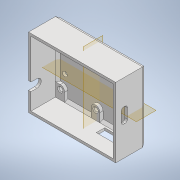
# Autodesk Inventor part: корпус
Saved by Autodesk Inventor 2021 (Build 250183000, 183)
## iProperties
Created: 2024-05-10
Part Number: корпус
Material: Типовые
Document SubType Name: Modeling
Designer: Мария
Density: 1 g/cm^3
Appearance: По умолчанию
Author: Мария
Autodesk Inventor part; units mm, degrees
ref_plane "YZ Plane" through (0, 0, 0) normal (1, 0, 0) x (0, 1, 0)
ref_plane "XZ Plane" through (0, 0, 0) normal (0, 1, 0) x (-1, 0, 0)
ref_plane "XY Plane" through (0, 0, 0) normal (0, 0, 1) x (1, 0, 0)
sketch "Эскиз1" plane through (0, 0, 0) normal (0, 0, 1) x (1, 0, 0)
  line L0 (2, 41.195) -> (54.5, 41.195) projected
  line L1 (54.5, 41.195) -> (54.5, 3.195) projected
  line L2 (0, 0) -> (56.5, 0)
  line L3 (56.5, 0) -> (56.5, 45.2)
  line L4 (56.5, 45.2) -> (0, 45.2)
  line L5 (0, 45.2) -> (0, 0)
  dimension "d0" = 52.5
  dimension "d1" = 38
  dimension "d2" = 56.5
  dimension "d3" = 45.2
  constraints: 8 end point, 2 parallel, 1 horizontal, 1 perpendicular
  measures "d0" distance of L0.start L0.end
  measures "d1" distance of L0.end L1.end
  measures "d2" distance of L3.end L4.end
  measures "d3" distance of L2.end L3.end
extrude "Выдавливание1" add sketch "Эскиз1" along normal blind 1.6
sketch "Эскиз2" plane through (0, 0, 1.6) normal (0, 0, 1) x (1, 0, 0)
  line L0 (56.5, 45.2) -> (0, 45.2) projected
  line L1 (0, 45.2) -> (0, 0) projected
  line L2 (56.5, 0) -> (56.5, 45.2) projected
  line L3 (0, 0) -> (56.5, 0) projected
  line L4 (1.6, 43.6) -> (54.9, 43.6)
  line L5 (54.9, 43.6) -> (54.9, 1.6)
  line L6 (54.9, 1.6) -> (1.6, 1.6)
  line L7 (1.6, 1.6) -> (1.6, 43.6)
  dimension "d6" = 1.6
  dimension "d7" = 1.6
  dimension "d8" = 1.6
  dimension "d9" = 1.6
  constraints: 8 end point, 2 parallel, 1 horizontal, 1 perpendicular
  measures "d6" distance between parallel lines of L0 L4
  measures "d7" distance between parallel lines of L1 L7
  measures "d8" distance between parallel lines of L3 L6
  measures "d9" distance between parallel lines of L2 L5
extrude "Выдавливание2" add sketch "Эскиз2" along normal blind 17.8
ref_plane "РабПлоскость1" through (0, 22.6, 0) normal (0, 1, 0) x (1, 0, 0)
ref_plane "РабПлоскость2" through (28.25, 0, 0) normal (1, 0, 0) x (0, 0, -1)
sketch "Эскиз3" plane through (0, 0, 0) normal (-1, 0, 0) x (0, 0, 1)
  circle A0 centre (15.47, 15.2304) radius 2.7
  line L0 (15.47, 17.9304) -> (19.4, 17.9304)
  line L1 (19.4, 1.6) -> (19.4, 43.6) projected
  line L2 (19.4, 17.9304) -> (19.4, 12.5304)
  line L3 (19.4, 12.5304) -> (15.47, 12.5304)
  line L4 (0, 0) -> (19.4, 0) projected
  circle A1 centre (15.27, 15.2304) radius 2.3 projected
  dimension "d39" = 5.4
  dimension "d41" = 3.93
  constraints: 6 end point, 2 point on circle, 2 point on line, 2 vertical alignment, 1 centre point, 1 horizontal, 1 horizontal alignment, 1 tangent
  measures "d39" diameter of A0
  measures "d41" distance from line of L2 A0.centre
extrude "Выдавливание3" cut sketch "Эскиз3" against normal up to surface (1.6 mm away) contours A0 | A0 L0 L1 L3 | A1
sketch "Эскиз4" plane through (54.9, 1.6, 1.6) normal (-1, 0, 0) x (0, 0, 1)
  line L0 (0, 0) -> (17.8, 0) projected
  line L1 (0, 0) -> (0, 42) projected
  line L2 (12.56, 18.055) -> (11.85, 18.055) projected
  line L3 (11.85, 17.905) -> (12.56, 17.905) projected
  line L4 (12.56, 18.055) -> (11.85, 18.055) projected
  line L5 (11.85, 17.905) -> (12.56, 17.905) projected
  arc A0 (12.56, 17.905) -> (13.81, 19.155) centre (12.56, 19.155) ccw projected
  line L6 (13.81, 19.155) -> (13.81, 25.595) projected
  arc A1 (10.6, 19.155) -> (11.85, 17.905) centre (11.85, 19.155) ccw projected
  line L7 (10.6, 25.595) -> (10.6, 19.155) projected
  arc A2 (11.85, 26.845) -> (10.6, 25.595) centre (11.85, 25.595) ccw projected
  line L8 (12.56, 26.845) -> (11.85, 26.845) projected
  arc A3 (13.81, 25.595) -> (12.56, 26.845) centre (12.56, 25.595) ccw projected
  line L9 (14.21, 25.595) -> (14.21, 19.155)
  arc A4 (12.56, 17.505) -> (14.21, 19.155) centre (12.56, 19.155) ccw
  line L10 (12.56, 17.505) -> (11.85, 17.505)
  arc A5 (10.2, 19.155) -> (11.85, 17.505) centre (11.85, 19.155) ccw
  line L11 (10.2, 19.155) -> (10.2, 25.595)
  arc A6 (11.85, 27.245) -> (10.2, 25.595) centre (11.85, 25.595) ccw
  line L12 (11.85, 27.245) -> (12.56, 27.245)
  arc A7 (14.21, 25.595) -> (12.56, 27.245) centre (12.56, 25.595) ccw
  point P0 (-1.6, -1.6)
  dimension "d50" = 1.65
  constraints: 8 end point, 8 point on circle, 8 tangent, 4 centre point, 3 parallel
  measures "d50" radius of A7
extrude "Выдавливание4" cut sketch "Эскиз4" against normal up to surface (1.6 mm away) contours A1 L7 A2 L8 A3 L6 A0 L3 | L9 A4 L10 A5 L11 A6 L12 A7
sketch "Эскиз5" plane through (0, 0, 0) normal (0, 0, -1) x (-1, 0, 0)
  circle A0 centre (-4.77, 37.84) radius 1.25
  circle A1 centre (-4.77, 7.36) radius 1.25
  circle A2 centre (-51.9, 37.84) radius 1.25
  circle A3 centre (-51.9, 7.36) radius 1.25
  circle A4 centre (-27.63, 37.84) radius 1.25
  circle A5 centre (-27.63, 7.36) radius 1.25
  line L0 (-56.5, 45.2) -> (0, 45.2) projected
  line L1 (0, 0) -> (-56.5, 0) projected
  line L2 (-28.25, -9.04) -> (-28.25, 54.24) projected
  line L3 (-56.5, 0) -> (-56.5, 45.2) projected
  line L4 (0, 45.2) -> (0, 0) projected
  dimension "d22" = 2.5
  dimension "d23" = 2.5
  dimension "d24" = 2.5
  dimension "d25" = 2.5
  dimension "d26" = 2.5
  dimension "d27" = 2.5
  dimension "d43" = 30.48
  dimension "d44" = 45.2
  dimension "d45" = 7.36
  dimension "d47" = 0.62
  dimension "d48" = 4.6
  dimension "d49" = 4.77
  constraints: 6 centre point, 4 horizontal alignment, 3 vertical alignment
  measures "d22" diameter of A2
  measures "d23" diameter of A4
  measures "d24" diameter of A0
  measures "d25" diameter of A3
  measures "d26" diameter of A5
  measures "d27" diameter of A1
  measures "d43" distance of A4.centre A5.centre
  measures "d44" distance between parallel lines of L0 L1
  measures "d45" distance from line of L1 A5.centre
  measures "d47" distance from line of L2 A5.centre
  measures "d48" distance from line of L3 A3.centre
  measures "d49" distance from line of L4 A1.centre
extrude "Выдавливание5" cut sketch "Эскиз5" against normal through all contours A0 | A1 | A2 | A3 | A4 L2 | L2 A4 | L2 A5 | A5 L2
sketch "Эскиз6" plane through (0, 0, 0) normal (0, -1, 0) x (1, 0, 0)
  line L0 (45.0915, 9.92) -> (35.1915, 9.92) projected
  line L1 (45.0915, 5.2) -> (45.0915, 9.92) projected
  line L2 (45.0915, 9.92) -> (35.1915, 9.92) projected
  line L3 (35.1915, 9.92) -> (35.1915, 5.2) projected
  line L4 (35.1915, 5.2) -> (45.0915, 5.2) projected
  line L5 (41.9515, 6.86) -> (41.9515, 6.9579) projected
  line L6 (40.3515, 6.86) -> (41.9515, 6.86) projected
  line L7 (38.3315, 6.86) -> (40.3515, 6.86) projected
  line L8 (38.3315, 8.26) -> (38.3315, 6.86) projected
  line L9 (40.3515, 8.26) -> (38.3315, 8.26) projected
  line L10 (41.9515, 8.26) -> (40.3515, 8.26) projected
  line L11 (41.9515, 8.1621) -> (41.9515, 8.26) projected
  line L12 (41.9515, 6.9579) -> (41.9515, 8.1621) projected
  line L13 (35.7915, 7.56) -> (36.5915, 6.76) projected
  line L14 (36.5915, 8.36) -> (35.7915, 7.56) projected
  line L15 (36.5915, 7.8267) -> (36.5915, 8.36) projected
  line L16 (37.1249, 7.8267) -> (36.5915, 7.8267) projected
  line L17 (37.1249, 7.2933) -> (37.1249, 7.8267) projected
  line L18 (36.5915, 7.2933) -> (37.1249, 7.2933) projected
  line L19 (36.5915, 6.76) -> (36.5915, 7.2933) projected
  line L20 (34.7915, 10.32) -> (45.4915, 10.32)
  line L21 (45.4915, 10.32) -> (45.4915, 4.8)
  line L22 (45.4915, 4.8) -> (34.7915, 4.8)
  line L23 (34.7915, 4.8) -> (34.7915, 10.32)
  point P0 (0, 0)
  dimension "d51" = 0.4
  dimension "d52" = 0.4
  dimension "d53" = 5.12
  dimension "d54" = 10.3
  constraints: 8 end point, 4 parallel
  measures "d51" distance between parallel lines of L1 L21
  measures "d52" distance between parallel lines of L0 L20
  measures "d53" distance between parallel lines of L0 L22
  measures "d54" distance between parallel lines of L1 L23
extrude "Выдавливание6" cut sketch "Эскиз6" against normal up to surface (1.6 mm away) contours L1 L4 L3 L0 | L6 L7 L8 L9 L10 L11 L12 L5 | L14 L15 L16 L17 L18 L19 L13 | L20 L21 L22 L23
fillet "Сопряжение1" [suppressed]
sketch "Эскиз7" plane through (0, 0, 1.6) normal (0, 0, 1) x (1, 0, 0)
  point P0 (0, 0)
sketch "Эскиз8" plane through (0, 0, 1.6) normal (0, 0, 1) x (1, 0, 0)
  circle A0 centre (4.77, 7.36) radius 1.25 projected
  circle A1 centre (51.9, 37.84) radius 1.25 projected
  line L0 (4.77, 7.36) -> (51.9, 7.36) construction
  line L1 (51.9, 7.36) -> (51.9, 37.84) construction
  line L2 (51.9, 37.84) -> (4.77, 37.84) construction
  line L3 (4.77, 37.84) -> (4.77, 7.36) construction
  line L4 (1.6, 1.6) -> (54.9, 1.6) projected
  line L5 (7.62, 1.6) -> (7.62, 7.36)
  line L6 (4.77, 10.21) -> (1.6, 10.21)
  line L7 (1.6, 43.6) -> (1.6, 1.6) projected
  line L8 (54.9, 43.6) -> (1.6, 43.6) projected
  line L9 (7.62, 43.6) -> (1.6, 43.6)
  line L10 (1.6, 43.6) -> (1.6, 34.99)
  line L11 (1.6, 34.99) -> (4.77, 34.99)
  line L12 (7.62, 37.84) -> (7.62, 43.6)
  line L13 (54.9, 1.6) -> (49.05, 1.6)
  line L14 (49.05, 1.6) -> (49.05, 7.36)
  line L15 (51.9, 10.21) -> (54.9, 10.21)
  line L16 (54.9, 10.21) -> (54.9, 1.6)
  line L17 (54.9, 1.6) -> (54.9, 43.6) projected
  line L18 (54.9, 43.6) -> (49.05, 43.6)
  line L19 (49.05, 43.6) -> (49.05, 37.84)
  line L20 (51.9, 34.99) -> (54.9, 34.99)
  line L21 (54.9, 34.99) -> (54.9, 43.6)
  line L22 (24.78, 43.6) -> (30.48, 43.6)
  line L23 (30.48, 43.6) -> (30.48, 37.84)
  line L24 (27.63, 34.99) -> (27.63, 34.99)
  line L25 (24.78, 37.84) -> (24.78, 43.6)
  line L26 (24.78, 1.6) -> (30.48, 1.6)
  line L27 (30.48, 1.6) -> (30.48, 7.36)
  line L28 (27.63, 10.21) -> (27.63, 10.21)
  line L29 (24.78, 7.36) -> (24.78, 1.6)
  circle A2 centre (27.63, 7.36) radius 1.25 projected
  circle A3 centre (27.63, 37.84) radius 1.25 projected
  arc A4 (7.62, 7.36) -> (4.77, 10.21) centre (4.77, 7.36) ccw
  arc A5 (4.77, 34.99) -> (7.62, 37.84) centre (4.77, 37.84) ccw
  arc A6 (27.63, 10.21) -> (24.78, 7.36) centre (27.63, 7.36) ccw
  arc A7 (30.48, 7.36) -> (27.63, 10.21) centre (27.63, 7.36) ccw
  arc A8 (24.78, 37.84) -> (27.63, 34.99) centre (27.63, 37.84) ccw
  arc A9 (27.63, 34.99) -> (30.48, 37.84) centre (27.63, 37.84) ccw
  arc A10 (51.9, 10.21) -> (49.05, 7.36) centre (51.9, 7.36) ccw
  arc A11 (49.05, 37.84) -> (51.9, 34.99) centre (51.9, 37.84) ccw
  circle A12 centre (51.9, 7.36) radius 1.25 projected
  circle A13 centre (4.77, 37.84) radius 1.25 projected
  point P0 (0, 0)
  point P1 (7.62, 10.21)
  point P2 (7.62, 34.99)
  point P3 (49.05, 34.99)
  point P4 (24.78, 34.99)
  point P5 (30.48, 10.21)
  point P6 (24.78, 10.21)
  point P7 (49.05, 1.6)
  point P8 (54.9, 34.99)
  point P9 (27.63, 10.21)
  point P10 (30.48, 1.6)
  dimension "d67" = 2.85
  constraints: 52 end point, 20 point on line, 16 point on circle, 16 tangent, 12 parallel, 9 coincident, 8 centre point, 8 perpendicular, 6 equal radius, 6 horizontal, 3 horizontal alignment
  measures "d67" radius of A11
extrude "Выдавливание7" add sketch "Эскиз8" along normal blind 2 contours L7 L6 A4 L5 L4 | L29 A6 A7 L27 L4 | L7 L8 L12 A5 L11 | L14 A10 L15 L16 L4 | L8 L23 A9 A8 L25 | L20 A11 L19 L8 L17
chamfer "Фаска1" distance 1.1547 angle 60 1 edges at (39.765, 43.6, 1.6) measured on face at (39.765, 43.1, 1.6)
chamfer "Фаска2" distance 1.1547 angle 60 5 edges at (16.2, 43.6, 1.6) (1.6, 22.6, 1.6) (16.2, 1.6, 1.6) (39.765, 1.6, 1.6) (54.9, 22.6, 1.6) measured on face at (2.1, 22.6, 1.6) measured on face at (54.4, 22.6, 1.6) measured on face at (16.2, 2.1, 1.6) measured on face at (16.2, 43.1, 1.6) measured on face at (39.765, 2.1, 1.6)
chamfer "Фаска3" [suppressed]
sketch "Эскиз9" plane through (0, 0, 0) normal (0, 0, -1) x (-1, 0, 0)
  line L0 (-56.5, 45.2) -> (0, 45.2) projected
  line L1 (-41.15, 45.2) -> (-15.35, 45.2)
  line L2 (-15.35, 45.2) -> (-15.35, 46.4)
  line L3 (-15.35, 46.4) -> (-41.15, 46.4)
  line L4 (-41.15, 46.4) -> (-41.15, 45.2)
  line L5 (-44.35, 45.2) -> (-12.15, 45.2)
  line L6 (-12.15, 45.2) -> (-12.15, 49.6)
  line L7 (-12.15, 49.6) -> (-44.35, 49.6)
  line L8 (-44.35, 49.6) -> (-44.35, 45.2)
  line L9 (0, 0) -> (-56.5, 0) projected
  line L10 (-41.15, 0) -> (-15.35, 0)
  line L11 (-15.35, 0) -> (-15.35, -1.2)
  line L12 (-15.35, -1.2) -> (-41.15, -1.2)
  line L13 (-41.15, -1.2) -> (-41.15, 0)
  line L14 (-44.35, 0) -> (-12.15, 0)
  line L15 (-12.15, 0) -> (-12.15, -4.4)
  line L16 (-12.15, -4.4) -> (-44.35, -4.4)
  line L17 (-44.35, -4.4) -> (-44.35, 0)
  line L18 (0, 45.2) -> (0, 0) projected
  line L19 (0, 6.5) -> (4.4, 6.5)
  line L20 (4.4, 6.5) -> (4.4, 38.7)
  line L21 (4.4, 38.7) -> (0, 38.7)
  line L22 (0, 38.7) -> (0, 6.5)
  line L23 (-56.5, 0) -> (-56.5, 45.2) projected
  line L24 (-56.5, 6.5) -> (-60.9, 6.5)
  line L25 (-60.9, 6.5) -> (-60.9, 38.7)
  line L26 (-60.9, 38.7) -> (-56.5, 38.7)
  line L27 (-56.5, 38.7) -> (-56.5, 6.5)
  line L28 (0, 9.7) -> (1.2, 9.7)
  line L29 (1.2, 9.7) -> (1.2, 35.5)
  line L30 (1.2, 35.5) -> (0, 35.5)
  line L31 (0, 35.5) -> (0, 9.7)
  line L32 (-56.5, 9.7) -> (-57.7, 9.7)
  line L33 (-57.7, 9.7) -> (-57.7, 35.5)
  line L34 (-57.7, 35.5) -> (-56.5, 35.5)
  line L35 (-56.5, 35.5) -> (-56.5, 9.7)
  point P0 (-28.25, 45.2)
  point P1 (-28.25, 46.4)
  point P2 (-28.25, -1.2)
  point P3 (-28.25, 0)
  point P4 (-28.25, -4.4)
  point P5 (-28.25, 49.6)
  point P6 (-28.25, 0)
  point P7 (-12.15, 0)
  point P8 (0, 22.6)
  point P9 (4.4, 22.6)
  point P10 (-60.9, 22.6)
  point P11 (-56.5, 22.6)
  point P12 (1.2, 22.6)
  point P13 (-56.5, 22.6)
  point P14 (0, 38.7)
  point P15 (0, 35.5)
  dimension "d79" = 1.2
  dimension "d80" = 3.2
  dimension "d81" = 3.2
  dimension "d82" = 25.8
  dimension "d83" = 25.8
  dimension "d84" = 3.2
  dimension "d85" = 3.2
  dimension "d86" = 1.2
  dimension "d116" = 25.8
  dimension "d117" = 3.2
  dimension "d118" = 1.2
  dimension "d119" = 3.2
  dimension "d123" = 3.2
  dimension "d124" = 3.2
  dimension "d125" = 1.2
  constraints: 64 end point, 16 parallel, 13 midpoint, 9 point on line, 8 horizontal, 8 perpendicular, 5 vertical alignment, 4 horizontal alignment
  measures "d79" distance between parallel lines of L0 L3
  measures "d80" distance between parallel lines of L3 L7
  measures "d81" horizontal distance of L2.end L5.end
  measures "d82" distance of L3.end L2.end
  measures "d83" distance between parallel lines of L13 L11
  measures "d84" distance between parallel lines of L16 L12
  measures "d85" distance between parallel lines of L15 L11
  measures "d86" distance between parallel lines of L10 L12
  measures "d116" distance of L32.end L33.end
  measures "d117" distance between parallel lines of L24 L32
  measures "d118" distance between parallel lines of L35 L33
  measures "d119" distance between parallel lines of L33 L25
  measures "d123" distance between parallel lines of L19 L28
  measures "d124" distance between parallel lines of L29 L20
  measures "d125" distance between parallel lines of L18 L29
extrude "Выдавливание8" [suppressed]
chamfer "Фаска13" [suppressed]
chamfer "Фаска14" [suppressed]
chamfer "Фаска15" [suppressed]
sketch "Эскиз11" plane through (0, 0, 1.6) normal (0, 0, 1) x (1, 0, 0)
  circle A0 centre (5.7547, 15.6) radius 1.5
  circle A1 centre (5.7547, 29.6) radius 1.5
  line L0 (2.7547, 10.21) -> (2.7547, 34.99) projected
  line L1 (-11.3, 22.6) -> (67.8, 22.6) projected
  point P0 (0, 0)
  dimension "d136" = 3
  dimension "d137" = 3
  dimension "d138" = 3
  dimension "d139" = 7
  dimension "d140" = 7
  constraints: 2 centre point, 1 vertical alignment
  measures "d136" diameter of A0
  measures "d137" diameter of A1
  measures "d138" distance from line of L0 A0.centre
  measures "d139" distance from line of L1 A0.centre
  measures "d140" distance from line of L1 A1.centre
extrude "Выдавливание9" cut sketch "Эскиз11" against normal through all
chamfer "Фаска16" distance 1.1547 angle 60 4 edges at (0, 22.6, 0) (28.25, 45.2, 0) (28.25, 0, 0) (56.5, 22.6, 0) measured on face at (28.25, 44.7, 0) measured on face at (56, 22.6, 0) measured on face at (0.5, 22.6, 0) measured on face at (28.25, 0.5, 0)
chamfer "Фаска17" distance 0.5 angle 45 6 edges at (3.52, 37.84, 3.6) (26.38, 37.84, 3.6) (50.65, 37.84, 3.6) (3.52, 7.36, 3.6) (26.38, 7.36, 3.6) (50.65, 7.36, 3.6)
equation "\"d7\" = d6"
equation "\"d8\" = d6"
equation "\"d9\" = d6"
equation "\"d23\" = d22"
equation "\"d24\" = d22"
equation "\"d25\" = d22"
equation "\"d26\" = d22"
equation "\"d27\" = d22"
equation "\"d45\" = -0.5 * d43 + 0.5 * d44"
equation "\"d83\" = d82"
equation "\"d84\" = d81"
equation "\"d85\" = d80"
equation "\"d86\" = d79"
equation "\"d119\" = d117"
equation "\"d123\" = d117"
equation "\"d124\" = d123"
equation "\"d125\" = d118"
equation "\"d140\" = d139"
